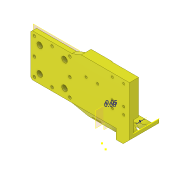
# Autodesk Inventor part: cellSTORM_v5_laserstage
Saved by Autodesk Inventor 2019.4 (Build 234330000, 330)
## iProperties
Created: 2020-04-25
Part Number: cellSTORM_v5_laserstage
Material: Generic
Document SubType Name: Modeling
Designer: diederichbenedict
Density: 1 g/cm^3
Appearance: Yellow
Author: diederichbenedict
Autodesk Inventor part; units mm, degrees
ref_plane "YZ Plane" through (0, 0, 0) normal (1, 0, 0) x (0, 1, 0)
ref_plane "XZ Plane" through (0, 0, 0) normal (0, 1, 0) x (-1, 0, 0)
ref_plane "XY Plane" through (0, 0, 0) normal (0, 0, 1) x (1, 0, 0)
ref_plane "Work Plane1" through (0, 0, 0) normal (0, 0, 1) x (1, 0, 0)
ref_plane "Work Plane2" through (-30, -30, 6) normal (0, 0, -1) x (0, 1, 0)
sketch "Sketch1" plane through (0, 0, 0) normal (0, 0, 1) x (1, 0, 0)
  circle A0 centre (-25, 0) radius 1.95 projected
  circle A1 centre (0, -25) radius 1.95 projected
  circle A2 centre (25, -25) radius 1.95 projected
  circle A3 centre (-25, 25) radius 1.95 projected
  circle A4 centre (25, 25) radius 1.95 projected
  circle A5 centre (-25, -25) radius 1.95 projected
  circle A6 centre (0, 25) radius 1.95 projected
  circle A7 centre (25, 0) radius 1.95 projected
  line L0 (-30, -28) -> (-28, -30) projected
  line L1 (-28, -30) -> (28, -30) projected
  line L2 (28, -30) -> (30, -28) projected
  line L3 (30, -28) -> (30, 28) projected
  line L4 (30, 28) -> (28, 30) projected
  line L5 (28, 30) -> (-28, 30) projected
  line L6 (-28, 30) -> (-30, 28) projected
  line L7 (-30, 28) -> (-30, -28) projected
  circle A8 centre (56, -8) radius 1.4 construction
  circle A9 centre (64, -8) radius 1.4 construction
  circle A10 centre (48, -8) radius 1.4 construction
  circle A11 centre (56, 20) radius 1.4 construction
  circle A12 centre (64, 20) radius 1.4 construction
  circle A13 centre (48, 20) radius 1.4 construction
  circle A14 centre (64, -18) radius 1.4 construction
  circle A15 centre (56, -18) radius 1.4 construction
  circle A16 centre (48, -18) radius 1.4 construction
  line L8 (40, 25) -> (72, 25) construction
  line L9 (40, 25) -> (40, -23) construction
  line L10 (72, -23) -> (40, -23) construction
  line L11 (72, 25) -> (72, -23) construction
  line L12 (66.4723, -44) -> (76, -44) projected
  line L13 (76, -44) -> (42, -44)
  line L14 (42, -44) -> (28, -30)
  line L15 (43, -44) -> (44, -44) projected
  arc A17 (49, 12.0684) -> (49, 10.4716) centre (47.85, 11.27) ccw
  arc A18 (63, 10.4716) -> (63, 12.0684) centre (64.15, 11.27) ccw
  circle A19 centre (47.85, 11.27) radius 1.6
  circle A20 centre (64.15, 11.27) radius 1.6
  line L16 (109, 34.77) -> (109, -13.23) construction
  line L17 (77, 34.77) -> (77, -13.23) construction
  line L18 (41.05, -13.23) -> (41.05, 35) construction
  line L19 (70.95, -13.23) -> (70.95, 35) construction
  line L20 (28, 30) -> (41.05, 35)
  line L21 (41.05, 35) -> (70.95, 35)
  line L22 (70.95, 35) -> (109, 35)
  line L23 (109, 35) -> (109, -13.23)
  line L24 (109, -13.23) -> (109, -44)
  line L25 (109, -44) -> (76, -44)
  arc A21 (85, -6.83) -> (85, -9.63) centre (85, -8.23) ccw
  arc A22 (85, 3.17) -> (85, 0.37) centre (85, 1.77) ccw
  arc A23 (85, 31.17) -> (85, 28.37) centre (85, 29.77) ccw
  arc A24 (101, 28.37) -> (101, 31.17) centre (101, 29.77) ccw
  arc A25 (101, 0.37) -> (101, 3.17) centre (101, 1.77) ccw
  arc A26 (101, -9.63) -> (101, -6.83) centre (101, -8.23) ccw
  circle A27 centre (85, -8.23) radius 1.6
  circle A28 centre (85, 1.77) radius 1.6
  circle A29 centre (85, 29.77) radius 1.6
  circle A30 centre (101, 29.77) radius 1.6
  circle A31 centre (101, 1.77) radius 1.6
  circle A32 centre (101, -8.23) radius 1.6
  point P0 (0, 0)
  dimension "d37" = 3.2
  dimension "d38" = 3.2
  dimension "d39" = 3.2
  dimension "d40" = 3.2
  dimension "d41" = 3.2
  dimension "d42" = 3.2
  dimension "d43" = 3.2
  dimension "d44" = 3.2
  constraints: 24 end point, 16 centre point, 16 point on circle, 8 coincident, 4 vertical, 3 horizontal, 2 perpendicular, 40 other
  measures "d37" diameter of A19
  measures "d38" diameter of A20
  measures "d39" diameter of A27
  measures "d40" diameter of A28
  measures "d41" diameter of A29
  measures "d42" diameter of A30
  measures "d43" diameter of A31
  measures "d44" diameter of A32
extrude "Extrusion1" add sketch "Sketch1" along normal up to surface (6 mm away)
sketch "Sketch2" plane through (-28, 30, 6) normal (0, 0, 1) x (1, 0, 0)
  circle A0 centre (10.5, -12.5) radius 1.95 projected
  circle A1 centre (10.5, -47.5) radius 1.95 projected
  circle A2 centre (45.5, -47.5) radius 1.95 projected
  circle A3 centre (45.5, -12.5) radius 1.95 projected
  point P0 (28, -30)
hole "Hole1" at (-17.5, -17.5, 6) at (17.5, -17.5, 6) at (17.5, 17.5, 6) at (-17.5, 17.5, 6) direction (0, 0, -1) diameter 4 end through all counterbore diameter 8 counterbore depth 4.5
sketch "Sketch4" plane through (0, 0, 0) normal (0, 0, -1) x (-1, 0, 0)
  line L0 (-28, -30) -> (-42, -44) projected
  line L1 (-42, -44) -> (-109, -44) projected
  line L2 (-109, -40) -> (-38, -40)
  line L3 (-72, -40) -> (-71.746, -39.8945)
  line L4 (-42, -44) -> (-109, -44) projected
  line L5 (-42, -44) -> (-109, -44)
  line L6 (-109, -44) -> (-108.9487, -40)
  line L7 (-75.5, -40) -> (-75.5, -44)
  point P0 (0, 0)
  dimension "d16" = 4
  constraints: 10 end point, 4 point on line, 2 horizontal, 1 midpoint, 1 parallel
  measures "d16" distance between parallel lines of L1 L2
extrude "Extrusion2" add sketch "Sketch4" along normal up to surface (35.7 mm away) contours L0 L1 L7 L2
sketch "Sketch6" plane through (42, -44, 6) normal (0, -1, 0) x (1, 0, 0)
  arc A0 (29.8555, -40.7) -> (30.8555, -41.7) centre (30.8555, -40.7) ccw construction
  line L0 (30.8555, -41.7) -> (34, -41.7) construction
  line L1 (34, -41.7) -> (34, -16) construction
  line L2 (34, -16) -> (24.4723, -16) construction
  arc A1 (24.4723, -16) -> (23.4723, -17) centre (24.4723, -17) ccw construction
  line L3 (23.4723, -17) -> (23.4723, -18.8624) construction
  arc A2 (22.4723, -19.8624) -> (23.4723, -18.8624) centre (22.4723, -18.8624) ccw construction
  line L4 (22.4723, -19.8624) -> (4, -19.8624) construction
  line L5 (4, -19.8624) -> (4, -31.397) construction
  arc A3 (3, -32.397) -> (4, -31.397) centre (3, -31.397) ccw construction
  line L6 (3, -32.397) -> (2, -32.397) construction
  arc A4 (2, -32.397) -> (1, -33.397) centre (2, -33.397) ccw construction
  line L7 (1, -33.397) -> (1, -35.9624) construction
  arc A5 (1, -35.9624) -> (2, -36.9624) centre (2, -35.9624) ccw construction
  line L8 (2, -36.9624) -> (28.8555, -36.9624) construction
  arc A6 (29.8555, -37.9624) -> (28.8555, -36.9624) centre (28.8555, -37.9624) ccw construction
  line L9 (29.8555, -37.9624) -> (29.8555, -40.7) construction
  line L10 (21.5, -35) -> (6, -35) construction
  line L11 (6, -35) -> (6, -21.5) construction
  line L12 (6, -21.5) -> (21.5, -21.5) construction
  line L13 (21.5, -21.5) -> (21.5, -35) construction
  circle A7 centre (31.5, -39) radius 1 construction
  circle A8 centre (25, -18.5) radius 1 construction
  circle A9 centre (3.5, -34) radius 1 construction
  line L14 (6, -21.5) -> (21.5, -21.5) construction
  line L15 (21.5, -25) -> (21.5, -35) construction
  line L16 (21.5, -35) -> (6, -35) construction
  line L17 (6, -35) -> (6, -25) construction
  line L18 (6, -21.5) -> (21.5, -21.5)
  line L19 (21.5, -25) -> (21.5, -35)
  line L20 (21.5, -35) -> (6, -35)
  line L21 (6, -35) -> (6, -25)
  circle A10 centre (25, -18.5) radius 1
  circle A11 centre (31.5, -39) radius 1
  circle A12 centre (3.5, -34) radius 1
  line L22 (5.1585, -25) -> (27.4978, -25)
  line L23 (27.4978, -25) -> (27.4978, -36.9624)
  line L24 (27.4978, -36.9624) -> (5.1585, -36.9624)
  line L25 (5.1585, -36.9624) -> (5.1585, -25)
  line L26 (0, 0) -> (67, 0) projected
  point P0 (-42, -6)
  dimension "d62" = 25
  constraints: 24 end point, 6 parallel, 3 centre point, 3 coincident, 3 concentric, 3 horizontal, 3 perpendicular, 3 point on line
  measures "d62" distance between parallel lines of L22 L26
extrude "Extrusion4" cut sketch "Sketch6" against normal through all
sketch "Sketch7" plane through (0, 0, 0) normal (0, 0, -1) x (-1, 0, 0)
  circle A0 centre (-64.15, 11.27) radius 1.6 projected
  circle A1 centre (-47.85, 11.27) radius 1.6 projected
  circle A2 centre (-101, -8.23) radius 1.6 projected
  circle A3 centre (-101, 1.77) radius 1.6 projected
  circle A4 centre (-85, 1.77) radius 1.6 projected
  circle A5 centre (-85, -8.23) radius 1.6 projected
  circle A6 centre (-85, 29.77) radius 1.6 projected
  circle A7 centre (-101, 29.77) radius 1.6 projected
  line L0 (-41.05, -13.23) -> (-41.05, 35)
  line L1 (-43.05, -13.23) -> (-49, -13.23)
  line L2 (-109, -44) -> (-109, 35) projected
  line L3 (-109, 35) -> (-41.05, 35)
  line L4 (-41.05, 35) -> (-41.05, -13.23)
  line L5 (-41.05, -13.23) -> (-109, -13.23)
  line L6 (-109, -13.23) -> (-109, 35)
  point P0 (0, 0)
  point P1 (-109, -13.23)
  constraints: 12 end point, 2 horizontal, 2 parallel, 1 perpendicular, 1 vertical, 4 other
ref_plane "Work Plane3" through (40, -23, -7) normal (0, 0, 1) x (1, 0, 0)
ref_plane "Work Plane4" through (107, -13.23, -7) normal (0, 0, 1) x (1, 0, 0)
extrude "Extrusion5" add sketch "Sketch7" along normal up to surface (7 mm away)
ref_plane "Work Plane8" through (72, -23, 6) normal (1, 0, 0) x (0, 0, -1)
sketch "Sketch8" plane through (72, -23, 6) normal (1, 0, 0) x (0, 0, -1)
  line L0 (0, -21) -> (0, 0) projected
  line L1 (41.7, -21) -> (0, -21) projected
  line L2 (41.7, -21) -> (41.7, -17) projected
  line L3 (41.7, -17) -> (13, 0) projected
  line L4 (13, 0) -> (6, 0) projected
  line L5 (6, 0) -> (0, 0) projected
  line L6 (-8, -7) -> (0, -7) projected
  line L7 (0, -7) -> (9.1538, -21)
  line L8 (41.7, -21) -> (0, -21) projected
  line L9 (0, -21) -> (9.1538, -21)
  line L10 (0, -21) -> (0, -7)
  line L11 (0, -7) -> (0, -21) projected
  line L12 (0, -21) -> (41.7, -21)
  line L13 (41.7, -21) -> (41.7, -23.7437)
  line L14 (41.7, -23.7437) -> (0, -23.7437)
  line L15 (0, -23.7437) -> (0, -21)
  point P0 (6, 23)
  constraints: 14 end point, 2 horizontal, 2 parallel, 2 perpendicular, 1 point on line
extrude "Extrusion6" cut sketch "Sketch8" along normal through all both and the other way through all contours L0 L7 L1 | L1 L13 L14 L15
sketch "Sketch9" plane through (109, -23, 0) normal (-1, 0, 0) x (0, 0, 1)
  line L0 (-0.5384, -17) -> (0, -16.1766) projected
  line L1 (0, -0.7484) -> (0, -16.1766) projected
  line L2 (0, -0.7484) -> (-7, -0.7484) projected
  line L3 (-7, -0.7484) -> (-17.6778, -7.0733) projected
  line L4 (-17.6778, -7.0733) -> (-17.6778, -8.2408) projected
  line L5 (-17.6778, -8.2408) -> (-19.6488, -8.2408) projected
  line L6 (-19.6488, -8.2408) -> (-34.4364, -17) projected
  line L7 (-0.5384, -17) -> (-34.4364, -17) projected
  line L8 (-0.5384, -17) -> (-34.4364, -17) projected
  line L9 (-4.1227, -17) -> (0, -10.6946)
  line L10 (0, -0.7484) -> (0, -16.1766) projected
  point P0 (0, 23)
  dimension "d29" = 3
  constraints: 2 end point, 2 point on line, 1 parallel
  measures "d29" distance between parallel lines of L9 L0
extrude "Extrusion7" add sketch "Sketch9" along normal up to surface from surface at 0 contours L7 L9 L1 L0 surface through (28, -30, 0) normal (-0.7071068, -0.7071068, 0)
sketch "Sketch10" plane through (0, 0, 0) normal (0, 0, -1) x (-1, 0, 0)
  circle A0 centre (-25, 25) radius 2.325 projected
  circle A1 centre (-25, -25) radius 2.325 projected
  circle A2 centre (25, 25) radius 2.325 projected
  circle A3 centre (25, -25) radius 2.325 projected
  circle A4 centre (25, -25) radius 2.325 projected
  point P0 (0, 0)
hole "Hole3" at (-25, 25, 0) at (25, 25, 0) at (-25, -25, 0) at (25, -25, 0) direction (0, 0, 1) diameter 3.8 depth 20 tip angle 118
sketch "Sketch11" plane through (109, -13.23, -7) normal (0, 0, -1) x (-1, 0, 0)
  line L0 (38.05, 0) -> (38.05, 48.23)
  line L1 (67.95, 0) -> (67.95, 48.23)
  line L2 (38.05, 48.23) -> (67.95, 48.23)
  line L3 (67.95, 48.23) -> (67.95, 0)
  line L4 (67.95, 0) -> (38.05, 0)
  line L5 (38.05, 0) -> (38.05, 48.23)
  circle A0 centre (44.85, 24.5) radius 1.6 projected
  circle A1 centre (61.15, 24.5) radius 1.6 projected
  point P0 (109, 13.23)
  constraints: 12 end point, 2 parallel, 2 vertical, 1 horizontal, 1 perpendicular, 4 other
extrude "Extrusion8" add sketch "Sketch11" along normal blind 0.8
sketch "Sketch12" plane through (0, 0, 0) normal (0, 0, -1) x (-1, 0, 0)
  line L0 (-59.5555, -27.9445) -> (-57.4342, -25.8231)
  line L1 (-54.323, -33.177) -> (-59.5555, -27.9445)
  line L2 (-57.4342, -25.8231) -> (-53.6158, -29.6415)
  line L3 (-53.6158, -29.6415) -> (-53.6158, -32.4699)
  line L4 (-53.6158, -32.4699) -> (-54.323, -33.177)
  line L5 (-54.323, -33.177) -> (-59.5555, -27.9445)
  line L6 (-75.5, -40) -> (-38, -40) projected
  line L7 (-62.5555, -40) -> (-50.6158, -40)
  line L8 (-50.6158, -40) -> (-50.6158, -24.8231)
  line L9 (-50.6158, -24.8231) -> (-62.5555, -24.8231)
  line L10 (-62.5555, -24.8231) -> (-62.5555, -40)
  point P0 (0, 0)
  point P1 (-75.2381, -40)
  point P2 (-108.9487, -40)
  dimension "d47" = 3
  dimension "d48" = 3
  dimension "d49" = 1
  constraints: 20 end point, 2 parallel, 1 horizontal, 1 perpendicular, 1 point on line, 1 vertical, 10 other
  measures "d47" distance from line of L10 L0.start
  measures "d48" distance between parallel lines of L8 L3
  measures "d49" distance from line of L0.end L9
ref_plane "Work Plane5" through (52.2016, -33.177, -19.05) normal (0, 0, 1) x (0.7071068, 0.7071068, 0)
extrude "Extrusion9" add sketch "Sketch12" along normal up to surface (19.05 mm away) contours L0 L2 L3 L4 L1 | L10 L9 L8 L6
sketch "Sketch13" plane through (62.5555, -40, -19.05) normal (0, 0, -1) x (-1, 0, 0)
  line L0 (0, 15.1769) -> (0, 0) projected
  line L1 (0, 0) -> (11.9397, 0) projected
  line L2 (11.9397, 0) -> (11.9397, 15.1769) projected
  line L3 (11.9397, 15.1769) -> (0, 15.1769) projected
  line L4 (3, 12.0555) -> (5.1213, 14.1769)
  line L5 (8.2326, 6.823) -> (3, 12.0555)
  line L6 (5.1213, 14.1769) -> (8.9397, 10.3585)
  line L7 (8.9397, 7.5301) -> (8.2326, 6.823)
  line L8 (8.9397, 10.3585) -> (8.9397, 7.5301)
  line L9 (8.2326, 6.823) -> (3, 12.0555)
  line L10 (8.2326, 6.823) -> (3, 12.0555)
  line L11 (2.9646, 12.0909) -> (5.1213, 14.2476)
  line L12 (5.1213, 14.2476) -> (8.9897, 10.3792)
  line L13 (8.9897, 10.3792) -> (8.9897, 7.5094)
  line L14 (8.9897, 7.5094) -> (8.2679, 6.7876)
  line L15 (8.176, 6.7664) -> (2.9434, 11.999)
  line L16 (2.9434, 11.999) -> (2.9081, 12.0343)
  line L17 (2.9081, 12.0343) -> (2.9646, 12.0909)
  line L18 (8.2679, 6.7876) -> (8.2114, 6.731)
  line L19 (8.2114, 6.731) -> (8.176, 6.7664)
  line L20 (11.9397, 15.1769) -> (0, 15.1769) projected
  line L21 (5.2782, 15.1769) -> (5.2782, 14.4044)
  line L22 (8.1383, 15.1769) -> (8.1383, 11.2306)
  line L23 (8.1383, 6.0359) -> (8.1383, 0)
  line L24 (4.2288, 10.7136) -> (0, 10.7136)
  line L25 (8.1383, 6.6579) -> (8.1383, 6.6579)
  line L26 (8.0044, 6.0359) -> (8.1383, 6.0359)
  line L27 (7.7561, 7.0401) -> (7.7561, 6.0359)
  line L28 (7.7561, 6.0359) -> (8.0185, 6.0359)
  line L29 (5.2782, 14.4044) -> (5.2782, 14.0907)
  line L30 (7.7561, 7.0401) -> (7.7561, 7.1863)
  point P0 (62.5555, 40)
  dimension "d52" = 0.05
  dimension "d53" = 0.08
  constraints: 52 end point, 15 point on line, 4 perpendicular, 4 vertical, 3 parallel, 2 collinear, 14 other
  measures "d52" distance between parallel lines of L4 L11
  measures "d53" distance between parallel lines of L5 L15
ref_plane "Work Plane6" through (52.2016, -33.177, -26.95) normal (0, 0, -1) x (-0.7071068, 0.7071068, 0)
chamfer "Chamfer1" distance 3 angle 45 2 edges at (50.6158, -40, -11.5614) (62.5555, -40, -11.5614)
ref_plane "Work Plane10" through (62.5555, -40, -15.5) normal (1, 0, 0) x (0, 0, -1)
ref_plane "Work Plane7" through (53.6158, -32.4699, -26.95) normal (-1, 0, 0) x (0, 0, 1)
ref_plane "Work Plane9" through (95.0506, -33.5506, -23) normal (0.7071068, -0.7071068, 0) x (0.7071068, 0.7071068, 0)
sketch "Sketch15" plane through (95.0506, -33.5506, -23) normal (0.7071068, -0.7071068, 0) x (0.7071068, 0.7071068, 0)
  circle A0 centre (0, 0) radius 5
  point P0 (-43.4871, 23)
  constraints: 1 centre point, 2 other
sketch "Sketch16" plane through (0, 0, 0) normal (0, 0, -1) x (-1, 0, 0)
  line L0 (-50.6158, -24.8231) -> (-50.6158, -33.6946) projected
  line L1 (-50.6158, -33.6946) -> (-31.6946, -33.6946) projected
  line L2 (-28, -30) -> (-31.6946, -33.6946) projected
  line L3 (28, -30) -> (-28, -30) projected
  line L4 (30, -28) -> (28, -30) projected
  line L5 (30, 28) -> (30, -28) projected
  line L6 (28, 30) -> (30, 28) projected
  line L7 (-28, 30) -> (28, 30) projected
  line L8 (-41.05, 35) -> (-28, 30) projected
  line L9 (-41.05, 35) -> (-41.05, -13.23) projected
  line L10 (-41.05, -13.23) -> (-109, -13.23) projected
  line L11 (-109, -33.6946) -> (-109, -13.23) projected
  line L12 (-109, -33.6946) -> (-62.5555, -33.6946) projected
  line L13 (-62.5555, -33.6946) -> (-62.5555, -24.8231) projected
  line L14 (-62.5555, -24.8231) -> (-50.6158, -24.8231) projected
  circle A0 centre (25, 0) radius 1.95 projected
  circle A1 centre (0, -25) radius 1.95 projected
  circle A2 centre (-25, -25) radius 1.95 projected
  circle A3 centre (25, 25) radius 1.95 projected
  circle A4 centre (-25, 25) radius 1.95 projected
  circle A5 centre (25, -25) radius 1.95 projected
  circle A6 centre (0, 25) radius 1.95 projected
  circle A7 centre (-25, 0) radius 1.95 projected
  circle A8 centre (17.5, 17.5) radius 2 projected
  circle A9 centre (-17.5, -17.5) radius 2 projected
  circle A10 centre (17.5, -17.5) radius 2 projected
  circle A11 centre (-17.5, 17.5) radius 2 projected
  line L15 (-42, -44) -> (-75.5, -44) projected
  line L16 (-109, -33.6946) -> (-109, -13.23) projected
  line L17 (-109, -27.3624) -> (-90.0667, -27.3624)
  line L18 (-90.0667, -27.3624) -> (-90.0667, -44)
  line L19 (-90.0667, -44) -> (-109, -44)
  line L20 (-109, -44) -> (-109, -27.3624)
  point P0 (0, 0)
  constraints: 8 end point, 2 parallel, 1 horizontal, 1 perpendicular, 1 point on line
extrude "Extrusion12" add sketch "Sketch16" against normal up to surface (6 mm away) contours L18 L19 L20 L12 | L12 L11 L17 L18
sketch "Sketch17" plane through (0, 0, 0) normal (0, 0, -1) x (-1, 0, 0)
  line L0 (9.6496, -138.2508) -> (-160.6256, 32.0244) projected
  line L1 (-109, -33.6946) -> (-109, -13.23) projected
  line L2 (-109, -29.5007) -> (-94.5007, -44)
  line L3 (-90.0667, -44) -> (-109, -44) projected
  line L4 (-100.1576, -44) -> (-109, -35.1576)
  line L5 (-109, -35.1576) -> (-109, -29.5007)
  line L6 (-100.1576, -44) -> (-98.7434, -45.4142)
  line L7 (-98.7434, -45.4142) -> (-93.0865, -45.4142)
  line L8 (-93.0865, -45.4142) -> (-94.5007, -44)
  line L9 (-93.0865, -45.4142) -> (-90.0667, -44)
  line L10 (-90.0667, -44) -> (-94.5007, -44)
  point P0 (0, 0)
  dimension "d66" = 7
  dimension "d67" = 4
  dimension "d86" = 2
  dimension "d87" = 135
  constraints: 16 end point, 3 parallel, 3 point on line, 1 collinear, 1 perpendicular
  measures "d66" distance between parallel lines of L2 L0
  measures "d67" distance between parallel lines of L2 L4
  measures "d86" distance of L4.start L6.end
  measures "d87" angle of L7 L6
extrude "Extrusion13" add sketch "Sketch17" along normal up to surface (35.7 mm away)
sketch "Sketch18" plane through (0, 0, 0) normal (0, 0, -1) x (-1, 0, 0)
  line L0 (-100.1576, -44) -> (-104.981, -39.1766) projected
  line L1 (-109, -39.1766) -> (-104.981, -39.1766) projected
  line L2 (-109, -44) -> (-109, -39.1766) projected
  line L3 (-100.1576, -44) -> (-109, -44) projected
  line L4 (-104.1576, -40) -> (-109, -35.1576) projected
  line L5 (-109, -35.1576) -> (-109, -40) projected
  line L6 (-109, -40) -> (-104.1576, -40) projected
  point P0 (0, 0)
extrude "Extrusion14" cut sketch "Sketch18" along normal through all both and the other way through all
sketch "Sketch19" plane through (75.5, -44, -35.7) normal (1, 0, 0) x (0, 0, -1)
  line L0 (-35.1616, 4) -> (-32.5462, 0) projected
  line L1 (-32.5462, 0) -> (0, 0) projected
  line L2 (0, 0) -> (0, 4) projected
  line L3 (-31.5773, 4) -> (0, 4) projected
  line L4 (-35.1616, 4) -> (-31.5773, 4) projected
  point P0 (-35.7, 44)
sketch "Sketch20" plane through (109, -29.5007, -35.7) normal (-0.7071068, 0.7071068, 0) x (-0.7071068, -0.7071068, 0)
  line L0 (14.8482, 35.1616) -> (13.6837, 35.7) projected
  line L1 (14.8482, 31.5773) -> (14.8482, 35.1616) projected
  line L2 (5.931, 35.7) -> (14.8482, 31.5773) projected
  line L3 (0, 35.7) -> (5.931, 35.7) projected
  line L4 (0, 35.7) -> (0, 0) projected
  line L5 (0, 0) -> (20.5051, 0) projected
  line L6 (20.5051, 35.7) -> (20.5051, 0) projected
  line L7 (13.6837, 35.7) -> (20.5051, 35.7) projected
  line L8 (14.8482, 31.5773) -> (14.8482, 0)
  line L9 (0, 0) -> (20.5051, 0) projected
  point P0 (56.2145, 35.7)
  constraints: 2 end point, 1 perpendicular, 1 point on line
extrude "Extrusion15" add sketch "Sketch19" along normal up to surface surface through (109, -35.1576, 0) normal (0.7071068, -0.7071068, 0)
sketch "Sketch21" plane through (95.0506, -33.5506, -23) normal (0.7071068, -0.7071068, 0) x (0.7071068, 0.7071068, 0)
  line L0 (-6.1405, 0.0323) -> (6.8595, 7.5379)
  line L1 (6.8595, 7.5379) -> (6.8595, -7.4732)
  line L2 (6.8595, -7.4732) -> (-6.1405, 0.0323)
  line L3 (-38.4252, 4) -> (-38.4252, -7.9624) projected
  line L4 (-41.2537, 4) -> (-38.4252, 4) projected
  line L5 (-41.2537, -7.9624) -> (-41.2537, 4) projected
  line L6 (-41.2537, -7.9624) -> (-38.4252, -7.9624) projected
  line L7 (-38.4252, 4) -> (-38.4252, -7.9624) projected
  point P0 (-43.4871, 23)
  point P1 (2.5262, 0.0323)
  dimension "d82" = 13
  constraints: 6 end point, 1 parallel, 7 other
  measures "d82" distance from line of L0.start L1
hole "Hole4" at (99.901, -28.7002, -30.4732) at (90.7086, -37.8926, -22.9677) at (99.901, -28.7002, -15.4621) direction (0.7071068, -0.7071068, 0) diameter 2.8 end through all counterbore diameter 7 counterbore depth 7
sketch "Sketch22" plane through (109, -29.5007, -35.7) normal (-0.7071068, 0.7071068, 0) x (-0.7071068, -0.7071068, 0)
  circle A0 centre (5.8679, 20.2379) radius 1.4 projected
  circle A1 centre (5.8679, 5.2268) radius 1.4 projected
  circle A2 centre (18.8679, 12.7323) radius 3.5 projected
  circle A3 centre (18.8679, 12.7323) radius 1.4 projected
  circle A4 centre (18.8679, 12.7323) radius 1.4 projected
  line L0 (18.8679, 12.7323) -> (5.8679, 5.2268)
  line L1 (5.8679, 5.2268) -> (5.8679, 20.2379)
  line L2 (5.8679, 20.2379) -> (18.8679, 12.7323)
  line L3 (23.1235, 11.0003) -> (5.2401, 0.6753)
  line L4 (2.2401, 2.4074) -> (2.2401, 23.0573)
  line L5 (5.2401, 24.7894) -> (23.1235, 14.4644)
  arc A5 (23.1235, 11.0003) -> (23.1235, 14.4644) centre (22.1235, 12.7323) ccw
  arc A6 (5.2401, 24.7894) -> (2.2401, 23.0573) centre (4.2401, 23.0573) ccw
  arc A7 (2.2401, 2.4074) -> (5.2401, 0.6753) centre (4.2401, 2.4074) ccw
  point P0 (56.2145, 35.7)
  point P1 (10.2012, 12.7323)
  dimension "d83" = 2
  constraints: 12 end point, 6 point on circle, 6 tangent, 3 centre point, 2 equal radius, 1 coincident, 9 other
  measures "d83" radius of A5
extrude "Extrusion16" cut sketch "Sketch22" along normal through all contours A0 L2 A2 L0 A1 L1 | L3 A7 L4 A6 L5 A5
body "Solid1"
